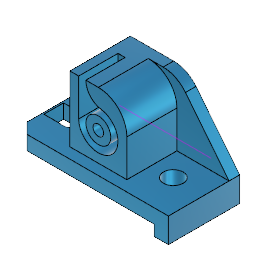
Z Belt Anchor R (Autodesk Fusion 360 design; units mm, degrees)
part number: Z Belt Anchor R
Autodesk Fusion 360 part; units mm, degrees
note: some values were not read from the file. Set by a fixed rule: which sketch regions a step uses.
sketch "Sketch7" plane through (0, 0, 27) normal (0, 0, 1) x (-1, 0, 0)
  circle A0 centre (-24.25, 0) radius 2.75
  line L0 (-46.25, 7) -> (-30.25, 7)
  line L1 (-30.25, 7) -> (-30.25, -10)
  line L2 (-30.25, -10) -> (-18.25, -10)
  line L3 (-18.25, -10) -> (-18.25, 10)
  line L4 (-18.25, 10) -> (-60.875, 10)
  line L5 (-24.25, -2.75) -> (-18.25, -2.75)
  line L6 (-18.25, 2.75) -> (-24.25, 2.75)
  line L7 (-18.75, -2.75) -> (-18.75, 2.75)
  circle A1 centre (-52.25, 0) radius 2.75
  line L8 (-60.875, 10) -> (-60.875, -7)
  line L9 (-60.875, -7) -> (-46.25, -7)
  line L10 (-46.25, -7) -> (-46.25, 7)
  dimension "d1" = 0.5
sketch "Sketch8" plane through (0, 7, 0) normal (0, 1, 0) x (-1, 0, 0)
  line L0 (-30.25, 23) -> (-56.875, 23)
  line L1 (-60.875, 27) -> (-46.25, 27)
  line L2 (-46.25, 45.3923) -> (-46.25, 27)
  line L3 (-34.75, 45.3923) -> (-46.25, 45.3923)
  arc A0 (-39.0357, 40.4436) -> (-34.75, 45.3923) centre (-39.75, 45.3923) ccw
  arc A1 (-39.0357, 40.4436) -> (-32.75, 35) centre (-38.25, 35) ccw
  line L4 (-32.75, 45.3923) -> (-32.75, 35)
  line L5 (-30.25, 45.3923) -> (-32.75, 45.3923)
  line L6 (-30.25, 45.3923) -> (-30.25, 23)
  line L7 (-46.25, 45.3923) -> (-30.25, 45.3923)
  line L8 (-46.25, 27) -> (-30.25, 27)
  line L9 (-46.25, 45.3923) -> (-60.875, 27)
  circle A2 centre (-38.25, 35) radius 1.5
  line L10 (-56.875, 20) -> (-56.875, 23)
  line L11 (-60.875, 20) -> (-56.875, 20)
  line L12 (-60.875, 27) -> (-60.875, 20)
sketch "Sketch9" plane through (0, -14, 0) normal (0, -1, 0) x (1, 0, 0)
  line L0 (27.125, 23) -> (56.875, 23)
  line L1 (29.4375, 0) -> (52.875, 0)
  line L2 (56.875, 4) -> (56.875, 23)
  line L3 (60.875, 45.3923) -> (60.875, 27)
  line L4 (20, 60.4011) -> (20, 94.0351)
  line L5 (20, 94.0351) -> (20.75, 94.0351)
  line L6 (20.75, 94.0351) -> (20.75, 23) construction
  circle A0 centre (26.75, 88.0351) radius 6
  line L7 (32.75, 88.0351) -> (32.75, 94.0351)
  line L8 (32.75, 94.0351) -> (34.75, 94.0351)
  line L9 (34.75, 94.0351) -> (34.75, 23) construction
  line L10 (32.75, 88.0351) -> (32.75, 23)
  circle A1 centre (38.25, 35) radius 3.5
  circle A2 centre (38.25, 35) radius 5.5
  arc A3 (34.75, 45.3923) -> (39.0357, 40.4436) centre (39.75, 45.3923) ccw
  line L11 (27.125, 45.3923) -> (60.875, 45.3923)
  line L12 (30.25, 45.3923) -> (30.25, 23)
  line L13 (60.875, 27) -> (46.25, 45.3923)
  line L14 (46.25, 45.3923) -> (46.25, 23)
  line L15 (20.75, 94.0351) -> (32.75, 94.0351) construction
  circle A4 centre (14, 60.4) radius 6
  line L16 (30.25, 23) -> (56.875, 23)
  line L17 (60.875, 27) -> (27.125, 27)
  line L18 (56.104, 33) -> (43.3735, 33) construction
  line L19 (46.25, 33) -> (34.8688, 27)
  circle A5 centre (38.25, 35) radius 1.5
  line L20 (52.875, 0) -> (56.875, 4)
  line L21 (0, 1) -> (1, 0)
  line L22 (0, 73.5) -> (13.1903, 73.5)
  line L23 (27.125, 23) -> (27.125, 60.4)
  arc A6 (27.125, 60.4) -> (14.8097, 73.5) centre (14, 60.4) ccw
  arc A7 (14.8097, 73.5) -> (13.1903, 73.5) centre (14, 60.4) ccw
  circle A8 centre (14, 60.4) radius 6
  line L24 (60.875, 27) -> (60.875, 20)
  line L25 (60.875, 20) -> (56.875, 20)
  line L26 (-3, 20) -> (56.875, 20)
  line L27 (-3, 73.5) -> (0, 73.5)
  line L28 (0, 1) -> (-3, 4)
  line L29 (-3, 4) -> (-3, 73.5)
  line L30 (26.9375, 3) -> (24.4375, 0)
  line L31 (29.4375, 0) -> (26.9375, 3)
  line L32 (1, 0) -> (24.4375, 0)
  dimension "d2" = 4
  dimension "d3" = 0.75
  dimension "d4" = 12
  dimension "d5" = 2
  dimension "d6" = 7
  dimension "d7" = 2
  dimension "d8" = 5
  dimension "d9" = 2.5
  dimension "d10" = 6.5
  dimension "d11" = 2.5
  dimension "d12" = 30.625
  dimension "d13" = 10
  dimension "d14" = 3
  dimension "d15" = 4
  measures "d4" diameter of A0
  measures "d6" diameter of A1
  measures "d7" distance of A1 A2
  measures "d8" radius of A3
  measures "d12" distance of origin
  measures "d14" diameter of A5
sketch "Sketch10" plane through (30.25, 0, 0) normal (-1, 0, 0) x (0, -1, 0)
  line L0 (7, 45.3923) -> (-10, 45.3923)
  line L1 (-10, 45.3923) -> (-10, 23)
  line L2 (7, 23) -> (7, 45.3923)
  line L3 (7, 23) -> (-10, 23)
  line L4 (7, 20) -> (-10, 20)
  line L5 (-10, 20) -> (-10, 27)
  line L6 (-10, 27) -> (-7, 27)
  line L7 (-7, 27) -> (7, 27)
  line L8 (7, 27) -> (7, 20)
sketch "Sketch11" plane through (0, -7, 0) normal (0, -1, 0) x (1, 0, 0)
  line L0 (30.25, 45.3923) -> (30.25, 27)
  line L1 (18.25, 27) -> (18.25, 23)
  line L2 (18.25, 23) -> (56.875, 23)
  line L3 (60.875, 27) -> (46.25, 27)
  line L4 (46.25, 27) -> (46.25, 45.3923)
  line L5 (46.25, 45.3923) -> (34.75, 45.3923)
  arc A0 (34.75, 45.3923) -> (39.0357, 40.4436) centre (39.75, 45.3923) ccw
  arc A1 (32.75, 35) -> (39.0357, 40.4436) centre (38.25, 35) ccw
  line L6 (32.75, 35) -> (32.75, 45.3923)
  line L7 (32.75, 45.3923) -> (30.25, 45.3923)
  line L8 (18.25, 27) -> (60.875, 27)
  circle A2 centre (10, 10) radius 2.75
  circle A3 centre (46.875, 10) radius 2.75
  line L9 (52.875, 27) -> (27.125, 27)
  line L10 (1, 0) -> (24.4375, 0)
  line L11 (52.875, 0) -> (56.875, 4)
  line L12 (56.875, 4) -> (56.875, 23)
  line L13 (30.25, 45.3923) -> (46.25, 45.3923)
  circle A4 centre (38.25, 35) radius 1.5
  circle A5 centre (38.25, 35) radius 3.5
  circle A6 centre (14, 60.4) radius 6
  line L14 (27.125, 27) -> (27.125, 60.4)
  arc A7 (27.125, 60.4) -> (13.1903, 73.5) centre (14, 60.4) ccw
  line L15 (13.1903, 73.5) -> (0, 73.5)
  line L16 (0, 1) -> (1, 0)
  line L17 (30.25, 27) -> (18.25, 27)
  line L18 (56.875, 23) -> (56.875, 20)
  line L19 (56.875, 20) -> (60.875, 20)
  line L20 (60.875, 20) -> (60.875, 27)
  line L21 (56.875, 23) -> (52.875, 27)
  line L22 (0, 73.5) -> (0, 1)
  line L23 (24.4375, 0) -> (26.9375, 3)
  line L24 (26.9375, 3) -> (29.4375, 0)
  line L25 (29.4375, 0) -> (52.875, 0)
extrude "Extrude1" add sketch "Sketch9" against normal blind 14 from surface at -7 contours L0 L10 L12 L16 L17 | L0 L10 L14 L16 L17 | L10 L11 L12 L17 | L0 L2 L14 L16 L17 L24 L25 | L10 A2 L17 L19 | L14 L17 L19 | A2 A3 L11 L14 L19 | A1 makes body 1 at (41.7326, 2.3333, 34.6515) makes body 2 at (39.125, -2.3333, 23)
extrude "Extrude5" add sketch "Sketch8" along normal blind 3 and the other way blind 3 bodies 1 2
extrude "Extrude11" cut 1 faces at (51.125, 4, 33.1308) along direction (0, 1, 0) blind 3 on bodies 1 bodies 1
extrude "Extrude6" add sketch "Sketch10" along normal blind 12 contours L1 L2 L3 L5 L6 L7 L8 bodies 1
hole "Hole1" at (52.25, 0, 27) direction (0, 0, -1) diameter 5.5 depth 10.5 tip angle 118 bodies 1
extrude "Extrude7" add sketch "Sketch11" along normal blind 3 contours L1 L2 L3 L8 L9 L17 L21 | L3 L8 L12 L18 L19 L20 L21 bodies 1
hole "Hole3" at (39.5625, 15.3125, 27) direction (0, 0, -1) diameter 5.5 depth 11 tip angle 118 bodies 1
extrude "Extrude9" cut sketch "Sketch7" against normal blind 8 contours A0 | A0 L5 L6 L7 bodies 1
chamfer "Chamfer1" distance 3 angle 45 2 edges at (18.25, -10, 25) (18.25, 10, 25) on bodies 1
fillet "Fillet1" radius 8 2 edges at (46.25, 0, 45.3923) (46.25, 8.5, 45.3923) on bodies 1
named bodies: "Z Belt Anchor R"
